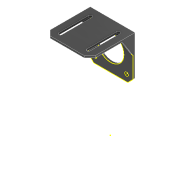
# Autodesk Inventor part: afirma_motor
Saved by Autodesk Inventor 2022 (Build 260153000, 153)
## iProperties
Created: 2022-11-14
Part Number: afirma_motor
Material: Generic
Document SubType Name: Modeling
Designer: ferna
Density: 1 g/cm^3
Appearance: Dark Gray
Author: ferna
Autodesk Inventor part; units mm, degrees
ref_plane "YZ Plane" through (0, 0, 0) normal (1, 0, 0) x (0, 1, 0)
ref_plane "XZ Plane" through (0, 0, 0) normal (0, 1, 0) x (-1, 0, 0)
ref_plane "XY Plane" through (0, 0, 0) normal (0, 0, 1) x (1, 0, 0)
sketch "Sketch1" plane through (0, 0, 0) normal (0, 0, 1) x (1, 0, 0)
  circle A0 centre (-23.2983, 91.6967) radius 2.75
  circle A1 centre (0, 115) radius 20
  circle A2 centre (23.9017, 91.6967) radius 2.75
  circle A3 centre (23.9017, 138.8967) radius 2.75
  circle A4 centre (-23.2983, 138.8967) radius 2.75
  line L0 (-23.2983, 91.6967) -> (-23.2983, 81.6967)
  line L1 (-23.2983, 81.6967) -> (-33.2983, 81.6967)
  line L2 (23.9017, 138.8967) -> (23.9017, 148.8967)
  line L3 (23.9017, 148.8967) -> (33.9017, 148.8967)
  line L4 (-25.2983, 81.6967) -> (25.9017, 81.6967)
  line L5 (33.9017, 89.6967) -> (33.9017, 148.8967)
  line L6 (33.9017, 148.8967) -> (-33.2983, 148.8967)
  line L7 (-33.2983, 148.8967) -> (-33.2983, 89.6967)
  line L8 (-33.2983, 89.6967) -> (-25.2983, 81.6967)
  line L9 (25.9017, 81.6967) -> (33.9017, 89.6967)
  point P0 (0, 0)
  point P1 (33.9017, 81.6967)
  dimension "d0" = 10
  dimension "d1" = 10
  dimension "d2" = 10
  dimension "d3" = 10
  dimension "d4" = 8
  dimension "d5" = 8
  dimension "d6" = 8
  dimension "d7" = 8
  constraints: 20 end point, 5 centre point, 4 point on line, 3 perpendicular, 2 parallel, 2 vertical, 1 horizontal
  measures "d0" distance of L0.start L0.end
  measures "d1" distance of L0.end L1.end
  measures "d2" distance of L2.start L2.end
  measures "d3" distance of L2.end L3.end
  measures "d4" distance of L7.end L1.end
  measures "d5" distance of L4.start L1.end
  measures "d6" distance of L4.end point (33.902, 81.697)
  measures "d7" distance of L5.start point (33.902, 81.697)
extrude "Extrusion1" add sketch "Sketch1" along normal blind 3
sketch "Sketch2" plane through (0, 0, 3) normal (0, 0, 1) x (1, 0, 0)
  line L0 (33.9017, 148.8967) -> (-33.2983, 148.8967) projected
  line L1 (33.9017, 89.6967) -> (33.9017, 148.8967) projected
  line L2 (-33.2983, 148.8967) -> (33.9017, 148.8967)
  line L3 (33.9017, 148.8967) -> (33.9017, 145.8967)
  line L4 (33.9017, 145.8967) -> (-33.2983, 145.8967)
  line L5 (-33.2983, 145.8967) -> (-33.2983, 148.8967)
  point P0 (0, 0)
  dimension "d10" = 3
  constraints: 8 end point, 2 parallel, 1 horizontal, 1 perpendicular, 1 point on line
  measures "d10" distance of L2.end L3.end
extrude "Extrusion2" add sketch "Sketch2" along normal blind 65
chamfer "Chamfer1" distance 8 angle 45 1 edges at (33.9017, 147.3967, 68)
chamfer "Chamfer2" distance 8 angle 45 1 edges at (-33.2983, 147.3967, 68)
sketch "Sketch3" plane through (-33.2983, 89.6967, 0) normal (-1, 0, 0) x (0, 0, 1)
  line L0 (3, 56.2) -> (60, 56.2) projected
  line L1 (3, 56.2) -> (3, 31.2)
  line L2 (3, 56.2) -> (3, 0) projected
  line L3 (3, 56.2) -> (19, 56.2)
  line L4 (19, 56.2) -> (3, 31.2)
  point P0 (0, -89.6967)
  dimension "d19" = 25
  dimension "d20" = 16
  constraints: 6 end point, 2 point on line
  measures "d19" distance of L0.start L1.end
  measures "d20" distance of L0.start L3.end
extrude "Extrusion3" add sketch "Sketch3" against normal blind 3
sketch "Sketch4" plane through (33.9017, 89.6967, 0) normal (1, 0, 0) x (0, 0, -1)
  line L0 (-19, 56.2) -> (-3, 56.2) projected
  line L1 (-19, 56.2) -> (-3, 31.2) projected
  line L2 (-3, 56.2) -> (-3, 31.2) projected
  point P0 (0, -89.6967)
extrude "Extrusion4" add sketch "Sketch4" against normal blind 3
sketch "Sketch5" plane through (-33.2983, 148.8967, 0) normal (0, 1, 0) x (1, 0, 0)
  line L0 (67.2, 0) -> (67.2, -60) projected
  line L1 (67.2, -60) -> (57.2, -60)
  line L2 (54.7, -60) -> (54.7, -60)
  line L3 (52.2, -57.5) -> (52.2, -12.5)
  line L4 (54.7, -10) -> (54.7, -10)
  line L5 (57.2, -12.5) -> (57.2, -57.5)
  line L6 (0, -19) -> (0, -60) projected
  line L7 (0, -60) -> (10, -60)
  line L8 (12.5, -60) -> (12.5, -60)
  line L9 (15, -57.5) -> (15, -12.5)
  line L10 (12.5, -10) -> (12.5, -10)
  line L11 (10, -12.5) -> (10, -57.5)
  arc A0 (12.5, -10) -> (10, -12.5) centre (12.5, -12.5) ccw
  arc A1 (15, -12.5) -> (12.5, -10) centre (12.5, -12.5) ccw
  arc A2 (12.5, -60) -> (15, -57.5) centre (12.5, -57.5) ccw
  arc A3 (10, -57.5) -> (12.5, -60) centre (12.5, -57.5) ccw
  arc A4 (52.2, -57.5) -> (54.7, -60) centre (54.7, -57.5) ccw
  arc A5 (54.7, -60) -> (57.2, -57.5) centre (54.7, -57.5) ccw
  arc A6 (57.2, -12.5) -> (54.7, -10) centre (54.7, -12.5) ccw
  arc A7 (54.7, -10) -> (52.2, -12.5) centre (54.7, -12.5) ccw
  point P0 (33.2983, 0)
  point P1 (52.2, -10)
  point P2 (52.2, -60)
  point P3 (57.2, -10)
  point P4 (15, -10)
  point P5 (10, -10)
  dimension "d25" = 10
  dimension "d26" = 5
  dimension "d27" = 50
  dimension "d28" = 10
  dimension "d29" = 5
  dimension "d30" = 2.5
  constraints: 20 end point, 16 point on circle, 16 tangent, 14 point on line, 8 centre point, 7 equal radius, 4 horizontal, 4 parallel, 2 perpendicular
  measures "d25" distance of L0.end L1.end
  measures "d26" distance of point (52.2, -10) point (57.2, -10)
  measures "d27" distance of point (52.2, -60) point (52.2, -10)
  measures "d28" distance of L6.end L7.end
  measures "d29" distance of point (10, -10) point (15, -10)
  measures "d30" radius of A0
extrude "Extrusion5" cut sketch "Sketch5" against normal through all
sketch "Sketch7" plane through (0, 0, 3) normal (0, 0, 1) x (1, 0, 0)
  line L0 (30.9017, 120.8967) -> (30.9017, 145.8967) projected
  line L1 (30.9017, 145.8967) -> (-30.2983, 145.8967) projected
  line L2 (-30.2983, 145.8967) -> (-30.2983, 120.8967) projected
  line L3 (-30.2983, 120.8967) -> (-33.2983, 120.8967) projected
  line L4 (-33.2983, 120.8967) -> (-33.2983, 89.6967) projected
  line L5 (-33.2983, 89.6967) -> (-25.2983, 81.6967) projected
  line L6 (-25.2983, 81.6967) -> (25.9017, 81.6967) projected
  line L7 (25.9017, 81.6967) -> (33.9017, 89.6967) projected
  line L8 (33.9017, 89.6967) -> (33.9017, 120.8967) projected
  line L9 (33.9017, 120.8967) -> (30.9017, 120.8967) projected
  circle A0 centre (0, 115) radius 20 projected
  circle A1 centre (-23.2983, 138.8967) radius 2.75 projected
  circle A2 centre (23.9017, 91.6967) radius 2.75 projected
  circle A3 centre (23.9017, 138.8967) radius 2.75 projected
  circle A4 centre (-23.2983, 91.6967) radius 2.75 projected
  point P0 (0, 0)
equation "\"d5\" = d4"
equation "\"d6\" = d4"
equation "\"d7\" = d6"
body "Solid1"
